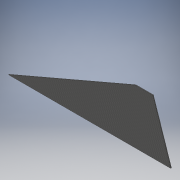
# Autodesk Inventor part: fin
Saved by Autodesk Inventor 2017 SP1 (Build 210196100, 196)
## iProperties
Created: 2016-10-22
Part Number: fin
Material: CFRP
Document SubType Name: Modeling
Designer: cflannery
Density: 1.43 g/cm^3
Appearance: Carbon Fiber
Author: cflannery
Autodesk Inventor part; units mm, degrees
ref_plane "YZ Plane" through (0, 0, 0) normal (1, 0, 0) x (0, 1, 0)
ref_plane "XZ Plane" through (0, 0, 0) normal (0, 1, 0) x (-1, 0, 0)
ref_plane "XY Plane" through (0, 0, 0) normal (0, 0, 1) x (1, 0, 0)
sketch "Sketch1" plane through (0, 0, 0) normal (0, 0, 1) x (1, 0, 0)
  line L0 (0, 0) -> (479.552, 205.486)
  line L1 (479.552, 205.486) -> (545.592, 205.486)
  line L2 (545.592, 205.486) -> (613.918, 0)
  line L3 (613.918, 0) -> (0, 0)
  dimension "d0" = 613.918
  dimension "d1" = 479.552
  dimension "d2" = 205.486
  dimension "d3" = 66.04
  constraints: 8 end point, 2 coincident, 1 horizontal, 1 parallel
  measures "d0" distance of L2.end L0.start
  measures "d1" horizontal distance of L0.end L0.start
  measures "d2" vertical distance of L1.end L2.end
  measures "d3" distance of L0.end L1.end
extrude "Extrusion1" add sketch "Sketch1" along normal blind 3.175
body "Solid1"
